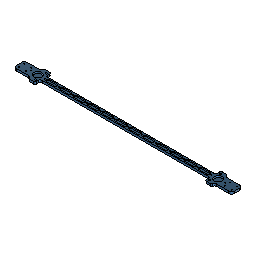
Mark3_final_printer_bridge (Autodesk Fusion 360 design; units mm, degrees)
Autodesk Fusion 360 part; units mm, degrees
sketch "Sketch1" plane through (0, 0, 0) normal (0, 1, 0) x (1, 0, 0)
sketch "Sketch2" plane through (0, 0, 0) normal (0, 1, 0) x (1, 0, 0)
  line L0 (472.4418, -33.5851) -> (472.4425, -33.5851)
  point P0 (-99.4552, -25.5851)
  point P1 (-99.4552, -10.5851)
  point P2 (-79.4552, -10.5851)
  point P3 (-79.4552, -25.5851)
  point P4 (514.3402, -10.5851)
  point P5 (514.3402, -25.5851)
  point P6 (494.3402, -25.5851)
  point P7 (494.3402, -10.5851)
  point P8 (-99.4552, -25.5851)
  point P9 (-79.4552, -25.5851)
  point P10 (-79.4552, -10.5851)
  point P11 (-99.4552, -10.5851)
  point P12 (514.3402, -10.5851)
  point P13 (514.3402, -25.5851)
  point P14 (494.3402, -25.5851)
  point P15 (494.3402, -10.5851)
  point P16 (-57.5575, -33.5851)
  point P17 (-57.5575, -2.5851)
  point P18 (472.4425, -33.5851)
  point P19 (472.4425, -3.0301)
  dimension "d4" = 15
  dimension "d5" = 20
  dimension "d6" = 15
  dimension "d7" = 20
  constraint coincident P8 P0
  constraint coincident P9 P3
  constraint coincident P10 P2
  constraint coincident P11 P1
  constraint coincident P12 P4
  constraint coincident P13 P5
  constraint coincident P14 P6
  constraint coincident P15 P7
  constraint coincident P18 L0.end
  measures "d4" distance of P8 P11
  measures "d5" distance of P8 P9
  measures "d6" distance of P14 P15
  measures "d7" distance of P13 P14
sketch "Sketch5" plane through (0, 0, 0) normal (0, -1, 0) x (1, 0, 0)
  circle A0 centre (514.3402, 10.5851) radius 1.5
  circle A1 centre (494.3402, 25.5851) radius 1.5
  circle A2 centre (514.3402, 25.5851) radius 1.5
  circle A3 centre (494.3402, 10.5851) radius 1.5
  circle A4 centre (-99.4552, 25.5851) radius 1.5
  circle A5 centre (-79.4552, 10.5851) radius 1.5
  circle A6 centre (-79.4552, 25.5851) radius 1.5
  circle A7 centre (-99.4552, 10.5851) radius 1.5
sketch "Sketch6" plane through (0, 0, 0) normal (0, 1, 0) x (1, 0, 0)
sketch "Sketch8" plane through (0, 0, 0) normal (0, 1, 0) x (1, 0, 0)
sketch "Sketch9" plane through (0, 0, 0) normal (0, 1, 0) x (1, 0, 0)
  point P0 (-57.5575, -33.5851)
  point P1 (472.4425, -33.5851)
sketch "Sketch10" plane through (0, 0, 0) normal (0, 1, 0) x (1, 0, 0)
sketch "Sketch11" plane through (0, 0, 0) normal (0, 1, 0) x (1, 0, 0)
sketch "Sketch12" plane through (0, 0, 0) normal (0, 1, 0) x (1, 0, 0)
  point P0 (-57.5575, -33.5851)
  point P1 (-57.5575, -2.5851)
sketch "Sketch13" plane through (0, 0, 0) normal (0, 1, 0) x (1, 0, 0)
  line L0 (-57.5575, -2.5851) -> (-98.8825, -2.5851)
  line L1 (-106.8825, -25.5851) -> (-106.8825, -10.5851)
  line L2 (-98.8825, -33.5851) -> (-57.5575, -33.5851)
  line L3 (472.4418, -33.5851) -> (513.7516, -33.5851)
  line L4 (472.4425, -3.0301) -> (513.7497, -3.0266)
  line L5 (521.7516, -25.5844) -> (521.7504, -11.0259)
  line L6 (472.4418, -33.5851) -> (472.4418, -36.5851)
  line L7 (-57.5575, -2.5851) -> (-57.5575, 0.4149)
  line L8 (-57.5575, -33.5851) -> (-57.5575, -36.5851)
  line L9 (-52.5575, 5.4149) -> (-42.5575, 5.4149)
  line L10 (467.4418, -41.5851) -> (457.4205, -41.5851)
  line L11 (472.4425, -3.0301) -> (472.4423, -0.0301)
  line L12 (467.4419, 4.9695) -> (457.4414, 4.9686)
  line L13 (-52.5575, -41.5851) -> (-42.5574, -41.5851)
  arc A0 (-106.8825, -25.5851) -> (-98.8825, -33.5851) centre (-98.8825, -25.5851) ccw
  arc A1 (-98.8825, -2.5851) -> (-106.8825, -10.5851) centre (-98.8825, -10.5851) ccw
  arc A2 (513.7516, -33.5851) -> (521.7516, -25.5844) centre (513.7516, -25.5851) ccw
  arc A3 (521.7504, -11.0259) -> (513.7497, -3.0266) centre (513.7504, -11.0266) ccw
  arc A4 (-57.5575, -36.5851) -> (-52.5575, -41.5851) centre (-52.5575, -36.5851) ccw
  arc A5 (-52.5575, 5.4149) -> (-57.5575, 0.4149) centre (-52.5575, 0.4149) ccw
  arc A6 (-42.5574, -41.5851) -> (-37.5574, -36.5851) centre (-42.5574, -36.5851) ccw
  arc A7 (-37.5575, 0.4149) -> (-42.5575, 5.4149) centre (-42.5575, 0.4149) ccw
  arc A8 (452.4205, -36.59) -> (457.4205, -41.5851) centre (457.4205, -36.5851) ccw
  arc A9 (467.4418, -41.5851) -> (472.4418, -36.5851) centre (467.4418, -36.5851) ccw
  arc A10 (457.4414, 4.9686) -> (452.4418, -0.0314) centre (457.4418, -0.0314) ccw
  arc A11 (472.4423, -0.0301) -> (467.4419, 4.9695) centre (467.4423, -0.0305) ccw
  circle A12 centre (458.355, -33.585) radius 2.5
  circle A13 centre (458.355, -2.585) radius 2.5
  circle A14 centre (-43.47, -33.585) radius 2.5
  circle A15 centre (-43.47, -2.585) radius 2.5
  line L14 (-37.5574, -29.0858) -> (-37.5574, -36.5851)
  line L15 (-37.5575, 0.4149) -> (-37.5575, -7.0849)
  line L16 (452.4095, -29.0795) -> (452.4205, -36.59)
  line L17 (452.4327, -7.0924) -> (452.4418, -0.0314)
  line L18 (447.4095, -24.0869) -> (-32.5574, -24.0858)
  line L19 (-32.5575, -12.0849) -> (447.4327, -12.086)
  arc A16 (447.4327, -12.086) -> (452.4327, -7.0924) centre (447.4327, -7.086) ccw
  arc A17 (452.4095, -29.0795) -> (447.4095, -24.0869) centre (447.4095, -29.0869) ccw
  arc A18 (-32.5574, -24.0858) -> (-37.5574, -29.0858) centre (-32.5574, -29.0858) ccw
  arc A19 (-37.5575, -7.0849) -> (-32.5575, -12.0849) centre (-32.5575, -7.0849) ccw
  line L20 (-32.5577, -18.1963) -> (-12.5577, -18.1963)
  line L21 (7.4423, -18.1964) -> (27.4423, -18.1964)
  line L22 (47.4423, -18.1964) -> (67.4423, -18.1965)
  line L23 (87.4423, -18.1965) -> (107.4423, -18.1965)
  line L24 (127.4423, -18.1965) -> (147.4423, -18.1966)
  line L25 (167.4423, -18.1966) -> (187.4423, -18.1966)
  line L26 (207.4423, -18.1966) -> (227.4423, -18.1967)
  line L27 (247.4423, -18.1967) -> (267.4423, -18.1967)
  line L28 (287.4423, -18.1967) -> (307.4423, -18.1968)
  line L29 (327.4423, -18.1968) -> (347.4423, -18.1968)
  line L30 (367.4423, -18.1968) -> (387.4423, -18.1969)
  line L31 (407.4423, -18.1968) -> (427.4423, -18.1969)
  line L32 (447.4423, -18.1969) -> (467.4423, -18.1969)
  line L33 (-72.5577, -18.1962) -> (-52.5577, -18.1962)
  line L34 (-23.9877, -22.9588) -> (-1.1277, -22.9589)
  arc A20 (-1.1277, -22.9589) -> (-1.1277, -13.4339) centre (-1.1277, -18.1964) ccw
  line L35 (-1.1277, -13.4339) -> (-23.9877, -13.4338)
  arc A21 (-23.9877, -13.4338) -> (-23.9877, -22.9588) centre (-23.9877, -18.1963) ccw
  line L36 (-23.9877, -18.1963) -> (-1.1277, -18.1964) construction
  point P0 (-43.47, -33.585)
  point P1 (-43.47, -2.585)
  point P2 (458.355, -33.585)
  point P3 (458.355, -2.585)
  point P4 (-57.5575, -33.5851)
  point P5 (-57.5575, -2.5851)
  point P6 (472.4418, -33.5851)
  point P7 (472.4425, -3.0301)
  point P8 (472.4418, -41.5851)
  point P9 (-57.5575, 5.4149)
  point P10 (-57.5575, -41.5851)
  point P11 (-37.5575, 5.4149)
  point P12 (452.4497, -41.5851)
  point P13 (472.4419, 4.9699)
  point P14 (452.4419, 4.9682)
  point P15 (-37.5575, -24.0851)
  point P16 (-37.5575, -12.0851)
  point P17 (452.4263, -24.0851)
  point P18 (452.4263, -12.0851)
  point P19 (207.4423, -18.1966)
  point P20 (487.4423, -18.1979)
  point P21 (447.4423, -18.1969)
  point P22 (407.4423, -18.1968)
  point P23 (367.4423, -18.1968)
  point P24 (327.4423, -18.1968)
  point P25 (287.4423, -18.1967)
  point P26 (247.4423, -18.1967)
  point P27 (167.4423, -18.1966)
  point P28 (127.4423, -18.1965)
  point P29 (87.4423, -18.1965)
  point P30 (47.4423, -18.1964)
  point P31 (7.4423, -18.1964)
  point P32 (-32.5577, -18.1963)
  point P33 (-72.5577, -18.1962)
  point P34 (-12.5577, -18.1963)
  point P35 (27.4423, -18.1964)
  point P36 (67.4423, -18.1965)
  point P37 (107.4423, -18.1965)
  point P38 (147.4423, -18.1966)
  point P39 (187.4423, -18.1966)
  point P40 (227.4423, -18.1967)
  point P41 (267.4423, -18.1967)
  point P42 (-52.5577, -18.1962)
  point P43 (307.4423, -18.1968)
  point P44 (347.4423, -18.1968)
  point P45 (387.4423, -18.1969)
  point P46 (427.4423, -18.1969)
  point P47 (467.4423, -18.1969)
  point P48 (-12.5577, -18.1963)
  point P49 (-12.5577, -18.1963)
  dimension "d73" = 501.825
  dimension "d82" = 8
  dimension "d83" = 8
  dimension "d84" = 8
  dimension "d86" = 20
  dimension "d88" = 8
  dimension "d89" = 20
  dimension "d91" = 8
  dimension "d92" = 5
  dimension "d93" = 5
  dimension "d94" = 5
  dimension "d95" = 5
  dimension "d96" = 5
  dimension "d97" = 5
  dimension "d98" = 5
  dimension "d99" = 5
  dimension "d100" = 5
  dimension "d101" = 5
  dimension "d102" = 5
  dimension "d148" = 5
  dimension "d151" = 40
  dimension "d152" = 40
  dimension "d153" = 40
  dimension "d154" = 40
  dimension "d155" = 40
  dimension "d156" = 40
  dimension "d157" = 40
  dimension "d158" = 40
  dimension "d159" = 40
  dimension "d160" = 40
  dimension "d161" = 40
  dimension "d162" = 40
  dimension "d163" = 40
  dimension "d164" = 40
  dimension "d173" = 20
  dimension "d174" = 20
  dimension "d175" = 20
  dimension "d176" = 20
  dimension "d177" = 20
  dimension "d178" = 20
  dimension "d179" = 20
  dimension "d180" = 20
  dimension "d181" = 20
  dimension "d182" = 20
  dimension "d183" = 20
  dimension "d184" = 20
  dimension "d185" = 20
  dimension "d186" = 20
  dimension "d197" = 9.525
  constraint coincident P5 L0.start
  constraint coincident P4 L2.end
  constraint perpendicular L1 L2
  constraint coincident P6 L3.start
  constraint coincident P7 L4.start
  constraint perpendicular L4 L5
  constraint perpendicular L3 L6
  constraint perpendicular L0 L7
  constraint perpendicular L2 L8
  constraint perpendicular L7 L9
  constraint perpendicular L6 L10
  constraint perpendicular L4 L11
  constraint perpendicular L11 L12
  constraint tangent L1 A0
  constraint tangent L2 A0
  constraint tangent L0 A1
  constraint tangent L1 A1
  constraint equal A0 A1
  constraint tangent L5 A2
  constraint tangent L3 A2
  constraint equal A0 A2
  constraint tangent L4 A3
  constraint tangent L5 A3
  constraint equal A0 A3
  constraint coincident P10 L8
  constraint coincident P10 L13
  constraint tangent L8 A4
  constraint tangent L13 A4
  constraint coincident P9 L7
  constraint coincident P9 L9
  constraint tangent L7 A5
  constraint tangent L9 A5
  constraint tangent L13 A6
  constraint coincident P11 L9
  constraint tangent L9 A7
  constraint coincident P12 L10
  constraint tangent L10 A8
  constraint coincident P8 L6
  constraint coincident P8 L10
  constraint tangent L6 A9
  constraint tangent L10 A9
  constraint coincident P14 L12
  constraint tangent L12 A10
  constraint coincident P13 L12
  constraint coincident P13 L11
  constraint tangent L12 A11
  constraint tangent L11 A11
  constraint equal A10 A11
  constraint coincident P2 A12.centre
  constraint coincident P3 A13.centre
  constraint coincident P0 A14.centre
  constraint coincident P1 A15.centre
  constraint tangent A6 L14
  constraint tangent A7 L15
  constraint parallel L18 L19
  constraint tangent L17 A16
  constraint tangent L19 A16
  constraint tangent L18 A17
  constraint tangent L16 A17
  constraint equal A16 A17
  constraint tangent L18 A18
  constraint tangent L14 A18
  constraint equal A16 A18
  constraint tangent L15 A19
  constraint tangent L19 A19
  constraint equal A16 A19
  constraint coincident P32 L20.start
  constraint parallel L19 L20
  constraint coincident P31 L21.start
  constraint parallel L18 L21
  constraint coincident P30 L22.start
  constraint parallel L18 L22
  constraint coincident P29 L23.start
  constraint parallel L18 L23
  constraint coincident P28 L24.start
  constraint parallel L18 L24
  constraint coincident P27 L25.start
  constraint parallel L18 L25
  constraint coincident P19 L26.start
  constraint parallel L18 L26
  constraint coincident P26 L27.start
  constraint parallel L18 L27
  constraint coincident P25 L28.start
  constraint parallel L18 L28
  constraint coincident P24 L29.start
  constraint parallel L19 L29
  constraint coincident P23 L30.start
  constraint parallel L18 L30
  constraint coincident P22 L31.start
  constraint parallel L19 L31
  constraint horizontal L32
  constraint coincident P21 L32.start
  constraint parallel L3 L32
  constraint coincident P33 L33.start
  constraint parallel L2 L33
  constraint coincident P49 P48
  constraint coincident P35 L21.end
  constraint coincident P36 L22.end
  constraint coincident P37 L23.end
  constraint coincident P38 L24.end
  constraint coincident P39 L25.end
  constraint coincident P40 L26.end
  constraint coincident P41 L27.end
  constraint coincident P42 L33.end
  constraint coincident P43 L28.end
  constraint coincident P44 L29.end
  constraint coincident P45 L30.end
  constraint coincident P46 L31.end
  constraint coincident P47 L32.end
  constraint tangent L34 A20
  constraint tangent A20 L35
  constraint parallel L34 L35
  constraint tangent L35 A21
  constraint tangent L34 A21
  constraint parallel L21 L36
  constraint midpoint L36 P49
  measures "d73" distance of P0 P2
  measures "d82" distance of P6 P8
  measures "d83" distance of P5 P9
  measures "d84" distance of P4 P10
  measures "d86" distance of P9 P11
  measures "d88" distance of P7 P13
  measures "d89" distance of P13 P14
  measures "d91" radius of A0
  measures "d92" radius of A4
  measures "d93" radius of A5
  measures "d94" radius of A6
  measures "d95" radius of A7
  measures "d96" radius of A8
  measures "d97" radius of A9
  measures "d98" radius of A10
  measures "d99" diameter of A12
  measures "d100" diameter of A13
  measures "d101" diameter of A14
  measures "d102" diameter of A15
  measures "d148" radius of A16
  measures "d151" distance of P19 P26
  measures "d152" distance of P25 P26
  measures "d153" distance of P24 P25
  measures "d154" distance of P23 P24
  measures "d155" distance of P22 P23
  measures "d156" distance of P21 P22
  measures "d157" distance of P19 P27
  measures "d158" distance of P27 P28
  measures "d159" distance of P28 P29
  measures "d160" distance of P29 P30
  measures "d161" distance of P30 P31
  measures "d162" distance of P31 P32
  measures "d163" distance of P32 P33
  measures "d164" distance of P20 P21
  measures "d173" distance of P32 P49
  measures "d174" distance of P31 P35
  measures "d175" distance of P30 P36
  measures "d176" distance of P29 P37
  measures "d177" distance of P28 P38
  measures "d178" distance of P27 P39
  measures "d179" distance of P19 P40
  measures "d180" distance of P26 P41
  measures "d181" distance of P25 P43
  measures "d182" distance of P24 P44
  measures "d183" distance of P23 P45
  measures "d184" distance of P22 P46
  measures "d185" distance of P21 P47
  measures "d186" distance of P33 P42
  measures "d197" diameter of A20
sketch "Sketch14" plane through (244.605, 0, 18.0851) normal (0, 1, 0) x (1, 0, 0)
sketch "Sketch15" plane through (0, 0, 0) normal (0, 1, 0) x (1, 0, 0)
sketch "Sketch22" plane through (0, 0, 0) normal (0, 1, 0) x (1, 0, 0)
sketch "Sketch23" plane through (0, 0, 0) normal (0, 1, 0) x (1, 0, 0)
sketch "Sketch24" plane through (0, 0, 0) normal (0, 1, 0) x (-1, 0, 0)
extrude "Extrude6" add sketch "Sketch13" along normal blind 6.35 contours L0 L1 L2 L3 L4 L5 L6 L7 L8 L9 L10 L11 L12 L13 A0 A1 A2 A3 A4 A5 A6 A7 A8 A9 A10 A11 L14 L15 L16 L17 L18 L19 A16 A17 A18 A19 | L34 A20 L35 A21 makes body 1
hole "Hole13" at (-32.5577, 0, 18.1963) at (7.4423, 0, 18.1964) at (47.4423, 0, 18.1964) at (87.4423, 0, 18.1965) at (127.4423, 0, 18.1965) at (167.4423, 0, 18.1966) at (207.4423, 0, 18.1966) at (247.4423, 0, 18.1967) at (287.4423, 0, 18.1967) at (327.4423, 0, 18.1968) at (367.4423, 0, 18.1968) at (407.4423, 0, 18.1968) at (447.4423, 0, 18.1969) at (487.4423, 0, 18.1979) at (-72.5577, 0, 18.1962) direction (0, 1, 0) diameter 3 depth 27.94 tip angle 118 bodies 1
hole "Hole14" at (514.3402, 0, 25.5851) at (514.3402, 0, 10.5851) at (494.3402, 0, 10.5851) at (494.3402, 0, 25.5851) at (-79.4552, 0, 10.5851) at (-79.4552, 0, 25.5851) at (-99.4552, 0, 25.5851) at (-99.4552, 0, 10.5851) direction (0, 1, 0) diameter 3 depth 27.94 tip angle 118 bodies 1
sketch "Sketch25" plane through (0, 0, 0) normal (0, 1, 0) x (1, 0, 0)
sketch "Sketch26" plane through (207.4347, 0, 18.0851) normal (0, 1, 0) x (1, 0, 0)
sketch "Sketch27" plane through (207.4347, 0, 18.0851) normal (0, 1, 0) x (1, 0, 0)
  point P0 (-260, 0)
  point P1 (-220, 0)
  point P2 (-180, 0)
  point P3 (-140, 0)
  point P4 (-100, 0)
  point P5 (-60, 0)
  point P6 (-20, 0)
  point P7 (20, 0)
  point P8 (60, 0)
  point P9 (100, 0)
  point P10 (140, 0)
  point P11 (180, 0)
  point P12 (220, 0)
  point P13 (260, 0)
  point P14 (260, 0)
  constraint coincident P13 P14
sketch "Sketch28" plane through (0, 0, 0) normal (0, 1, 0) x (1, 0, 0)
move_face "OffsetFaces1" offset 1.9367 2 faces at (287.4206, 2.1167, 24.0865) (127.4392, 2.1167, 12.0852) on bodies 1
sketch "Sketch29" plane through (0, 0, 0) normal (0, 1, 0) x (1, 0, 0)
sketch "Sketch30" plane through (0, 0, 0) normal (0, 1, 0) x (1, 0, 0)
fillet "Fillet3" radius 6.35 4 edges at (-57.5575, 3.175, 33.5851) (-57.5575, 3.175, 2.5851) (472.4425, 3.175, 3.0301) (472.4418, 3.175, 33.5851) on bodies 1
hole "Hole15" at (-52.5577, 0, 18.1962) direction (0, 1, 0) diameter 22.225 depth 5.08 tip angle 180 bodies 1
hole "Hole16" at (467.4423, 0, 18.1969) direction (0, 1, 0) diameter 22.225 depth 5.08 tip angle 180 bodies 1
sketch "Sketch31" plane through (0, 0, 0) normal (0, 1, 0) x (1, 0, 0)
extrude "Extrude7" add sketch "Sketch13" along normal blind 3.81 separate body contours L34 A20 L35 A21 makes body 2
copy_body "CopyPasteBodies5" bodies 2 makes body 3
copy_body "CopyPasteBodies6" bodies 2 makes body 4
move_body "Move7" bodies 4 to x (1, 0, 0) y (0, 1, 0) z (0, 0, 1) at (40, 0, 0)
copy_body "CopyPasteBodies7" bodies 2 makes body 5
move_body "Move8" bodies 5 to x (1, 0, 0) y (0, 1, 0) z (0, 0, 1) at (80, 0, 0)
copy_body "CopyPasteBodies8" bodies 2 makes body 6
move_body "Move9" bodies 6 to x (1, 0, 0) y (0, 1, 0) z (0, 0, 1) at (120, 0, 0)
copy_body "CopyPasteBodies9" bodies 2 makes body 7
move_body "Move10" bodies 7 to x (1, 0, 0) y (0, 1, 0) z (0, 0, 1) at (160, 0, 0)
copy_body "CopyPasteBodies10" bodies 2 makes body 8
move_body "Move11" bodies 8 to x (1, 0, 0) y (0, 1, 0) z (0, 0, 1) at (200, 0, 0)
copy_body "CopyPasteBodies11" bodies 2 makes body 9
move_body "Move12" bodies 9 to x (1, 0, 0) y (0, 1, 0) z (0, 0, 1) at (240, 0, 0)
copy_body "CopyPasteBodies12" bodies 2 makes body 10
move_body "Move13" bodies 10 to x (1, 0, 0) y (0, 1, 0) z (0, 0, 1) at (280, 0, 0)
copy_body "CopyPasteBodies13" bodies 2 makes body 11
move_body "Move14" bodies 11 to x (1, 0, 0) y (0, 1, 0) z (0, 0, 1) at (320, 0, 0)
copy_body "CopyPasteBodies14" bodies 2 makes body 12
move_body "Move15" bodies 12 to x (1, 0, 0) y (0, 1, 0) z (0, 0, 1) at (360, 0, 0)
copy_body "CopyPasteBodies15" bodies 2 makes body 13
move_body "Move16" bodies 13 to x (1, 0, 0) y (0, 1, 0) z (0, 0, 1) at (400, 0, 0)
copy_body "CopyPasteBodies16" bodies 2 makes body 14
move_body "Move17" bodies 14 to x (1, 0, 0) y (0, 1, 0) z (0, 0, 1) at (440, 0, 0)
copy_body "CopyPasteBodies19" bodies 5 makes body 15
move_body "Move18" bodies 15 to x (1, 0, 0) y (0, 1, 0) z (0, 0, 1) at (-40, 0, 0)
combine "Combine2" operation cut target body 1 tool bodies 2 4 6 7 8 9 10 11 12 13 14
combine "Combine3" operation cut target body 1 tool bodies 3
copy_body "CopyPasteBodies17" bodies 2
copy_body "CopyPasteBodies18" bodies 2
combine "Combine4" operation cut target body 1 tool bodies 5 15
move_body "Move19" bodies 1 to x (1, 0, 0) y (0, 0, -1) z (0, 1, 0) at (0, 5.4149, -5.4149)
